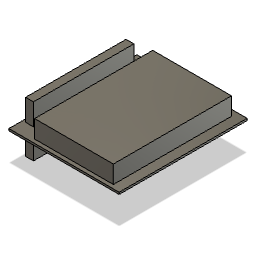
Battery Hat (Autodesk Fusion 360 design; units mm, degrees)
Autodesk Fusion 360 part; units mm, degrees
sketch "Sketch1" plane through (0, 0, 0) normal (0, 1, 0) x (1, 0, 0)
  line L0 (0, 0) -> (56, 0)
  line L1 (56, 0) -> (56, -65)
  line L2 (56, -65) -> (0, -65)
  line L3 (0, -65) -> (0, 0)
  dimension "d1" = 56
  dimension "d2" = 65
  constraint horizontal L0
  constraint vertical L1
  constraint horizontal L2
  constraint vertical L3
  constraint coincident L0.start L3.end
  measures "d1" distance of L0.start L0.end
  measures "d2" distance of L0.start L2.end
extrude "Extrude1" add sketch "Sketch1" along normal blind 1
sketch "Sketch2" plane through (0, 1, 0) normal (0, 1, 0) x (-1, 0, 0)
  line L0 (0, 65) -> (-56, 65)
  line L1 (-56, 65) -> (-56, 0)
  line L2 (-56, 0) -> (0, 0)
  line L3 (0, 0) -> (0, 65)
  line L4 (-1.5, 7) -> (-5.5, 7)
  line L5 (-5.5, 7) -> (-5.5, 58)
  line L6 (-5.5, 58) -> (-1.5, 58)
  line L7 (-1.5, 58) -> (-1.5, 7)
  dimension "d5" = 4
  dimension "d6" = 51
  dimension "d7" = 7
  dimension "d8" = 7
  dimension "d9" = 1.5
  constraint horizontal L4
  constraint vertical L5
  constraint horizontal L6
  constraint vertical L7
  measures "d5" distance of L4.start L4.end
  measures "d6" distance of L4.start L6.end
  measures "d7" distance of L2 L4
  measures "d8" distance of L0 L6
  measures "d9" distance of L3 L7
extrude "Extrude2" add sketch "Sketch2" along normal blind 11 contours L4 L5 L6 L7
sketch "Sketch3" plane through (0, 0, 0) normal (0, -1, 0) x (1, 0, 0)
  line L0 (56, 65) -> (0, 65)
  line L1 (0, 65) -> (0, 0)
  line L2 (0, 0) -> (56, 0)
  line L3 (56, 0) -> (56, 65)
  line L4 (1.5, 7) -> (5.5, 7)
  line L5 (5.5, 7) -> (5.5, 58)
  line L6 (5.5, 58) -> (1.5, 58)
  line L7 (1.5, 58) -> (1.5, 7)
  constraint horizontal L4
  constraint vertical L5
  constraint horizontal L6
  constraint vertical L7
extrude "Extrude3" add sketch "Sketch3" along normal blind 14 contours L4 L5 L6 L7
sketch "Sketch4" plane through (0, 1, 0) normal (0, 1, 0) x (-1, 0, 0)
  line L0 (-1.5, 58) -> (-1.5, 7)
  line L1 (-1.5, 7) -> (-5.5, 7)
  line L2 (-5.5, 7) -> (-5.5, 58)
  line L3 (-5.5, 58) -> (-1.5, 58)
  line L4 (0, 65) -> (-56, 65)
  line L5 (-56, 65) -> (-56, 0)
  line L6 (-56, 0) -> (0, 0)
  line L7 (0, 0) -> (0, 65)
  line L8 (-11.1237, 3.0691) -> (-51.1237, 3.0691)
  line L9 (-51.1237, 3.0691) -> (-51.1237, 63.0691)
  line L10 (-51.1237, 63.0691) -> (-11.1237, 63.0691)
  line L11 (-11.1237, 63.0691) -> (-11.1237, 3.0691)
  dimension "d14" = 40
  dimension "d15" = 60
  constraint horizontal L8
  constraint vertical L9
  constraint horizontal L10
  constraint vertical L11
  measures "d14" distance of L8.start L8.end
  measures "d15" distance of L8.start L10.end
extrude "Extrude4" add sketch "Sketch4" along normal blind 9 contours L8 L9 L10 L11
